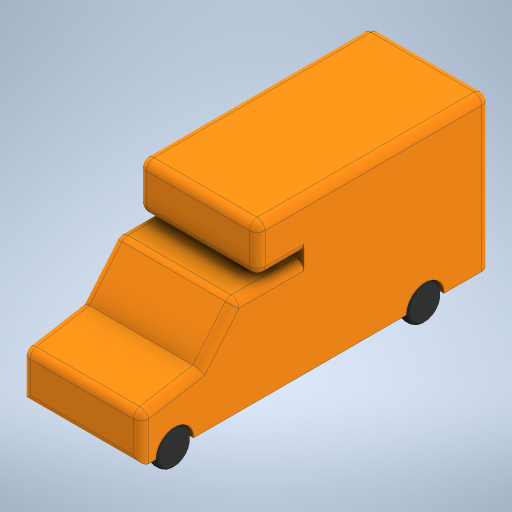
# Autodesk Inventor part: BungaCamp-Uhaul15ft
Saved by Autodesk Inventor 2023 (Build 270158000, 158)
## iProperties
Created: 2024-07-15
Part Number: BungaCamp-Uhaul15ft
Material: Generic
Document SubType Name: Modeling
Designer: incep
Density: 1 g/cm^3
Appearance: Default
Author: incep
Autodesk Inventor part; units mm, degrees
ref_plane "YZ Plane" through (0, 0, 0) normal (1, 0, 0) x (0, 1, 0)
ref_plane "XZ Plane" through (0, 0, 0) normal (0, 1, 0) x (-1, 0, 0)
ref_plane "XY Plane" through (0, 0, 0) normal (0, 0, 1) x (1, 0, 0)
sketch "Sketch4" plane through (0, 0, 0) normal (1, 0, 0) x (0, 1, 0)
  line L0 (2980.85, 1828.8) -> (0, 1828.8)
  line L1 (0, 1828.8) -> (0, -1828.8)
  line L2 (0, -1828.8) -> (2980.85, -1828.8)
  line L3 (2980.85, -1828.8) -> (2980.85, 1828.8)
  line L4 (2980.85, 2743.2) -> (2066.45, 2743.2)
  line L5 (2066.45, 2743.2) -> (2066.45, 1828.8)
  line L6 (2066.45, 1828.8) -> (2980.85, 1828.8)
  line L7 (2980.85, 1828.8) -> (2980.85, 2743.2)
  circle A0 centre (0, -558.8) radius 371.95
  line L8 (-371.95, 34.5004) -> (-371.95, -1152.1004) construction
  line L9 (0, 1828.8) -> (1914.05, 1828.8)
  line L10 (1914.05, 1828.8) -> (1914.05, 3174.9998)
  line L11 (1914.05, 3174.9998) -> (1096.7454, 3860.7998)
  line L12 (890.7249, 5029.1998) -> (1.7249, 5029.1998)
  line L13 (890.7249, 5029.1998) -> (1096.7454, 3860.7998)
  circle A1 centre (1.369, 4368.7999) radius 371.95
  line L14 (0, 1828.8) -> (1.7249, 5029.1998)
  point P0 (0, 0)
  point P1 (0, 0)
  point P2 (-371.95, -558.8)
  point P3 (1.5695, 4740.7498)
  point P4 (1.1685, 3996.8499)
  point P5 (0, -186.85)
  point P6 (0, -930.75)
  dimension "d2" = 4572
  dimension "d3" = 914.4
  dimension "d4" = 743.9
  dimension "d5" = 3352.8
  dimension "d6" = 914.4
  dimension "d7" = 6858
  dimension "d8" = 660.4
  dimension "d9" = 1270
  dimension "d10" = 152.4
  dimension "d11" = 130
  dimension "d12" = 100
  dimension "d13" = 889
  dimension "d14" = 685.8
  dimension "d15" = 1168.4
  constraints: 30 end point, 4 parallel, 3 horizontal, 2 centre point, 2 collinear, 2 midpoint, 2 perpendicular, 2 point on line, 1 coincident, 1 equal radius, 1 horizontal alignment, 1 tangent, 1 vertical
  measures "d2" distance between parallel lines of L2 L4
  measures "d3" distance of L4.start L4.end
  measures "d4" diameter of A0
  measures "d5" distance between parallel lines of L3 L8
  measures "d6" distance of L4.end L5.end
  measures "d7" distance of L1.end L12.end
  measures "d8" distance of A1.centre L12.end
  measures "d9" distance of L1.end A0.centre
  measures "d10" distance between parallel lines of L5 L10
  measures "d11" angle of L10 L11
  measures "d12" angle of L12 L13
  measures "d13" distance of L12.start L12.end
  measures "d14" vertical distance of L10.end L11.end
  measures "d15" vertical distance of L11.end L12.start
extrude "Extrusion1" add sketch "Sketch4" along normal mid plane 2336.8 contours L3 L2 L1 A0 L0 | L0 L5 L4 L7 | L0 L14 A1 L12 L13 L11 L10
sketch "Sketch5" plane through (1168.4, 0, 0) normal (1, 0, 0) x (0, 0, -1)
  circle A0 centre (-4368.7999, 1.369) radius 371.95 projected
  circle A1 centre (558.8, 0) radius 371.95 projected
  circle A2 centre (-4368.7999, 1.369) radius 346.55
  circle A3 centre (558.8, 0) radius 346.55
  point P0 (0, 0)
  dimension "d18" = 25.4
  dimension "d19" = 25.4
  constraints: 2 centre point
  measures "d18" radial gap between concentric circles of A0 A2
  measures "d19" radial gap between concentric circles of A1 A3
extrude "Extrusion2" add sketch "Sketch5" against normal blind 225 contours A2 | A3
sketch "Sketch6" plane through (-1168.4, 0, 0) normal (-1, 0, 0) x (0, 0, 1)
  circle A0 centre (-558.8, 0) radius 371.95 projected
  circle A1 centre (4368.7999, 1.369) radius 371.95 projected
  circle A2 centre (-558.8, 0) radius 346.55
  circle A3 centre (4368.7999, 1.369) radius 346.55
  point P0 (0, 0)
  dimension "d22" = 25.4
  dimension "d23" = 25.4
  constraints: 2 centre point
  measures "d22" radial gap between concentric circles of A0 A2
  measures "d23" radial gap between concentric circles of A1 A3
extrude "Extrusion3" add sketch "Sketch6" against normal blind 225 contours A2 | A3
fillet "Fillet1" radius 152.4 22 edges at (1168.4, 446.2249, 5029.1998) (-1168.4, 446.2249, 5029.1998) (-1168.4, 993.7352, 4444.9998) (1168.4, 993.7352, 4444.9998) (1168.4, 1505.3977, 3517.8998) (-1168.4, 1505.3977, 3517.8998) (0, 1914.05, 3174.9998) (1168.4, 2523.65, 2743.2) (-1168.4, 2523.65, 2743.2) (0, 2980.85, 2743.2) (0, 2066.45, 2743.2) (1168.4, 1914.05, 2501.8999) (-1168.4, 1914.05, 2501.8999) (0, 890.7249, 5029.1998) (1168.4, 2980.85, 457.2) (0, 2980.85, -1828.8) (-1168.4, 2980.85, 457.2) (1168.4, 1490.425, -1828.8) (-1168.4, 1490.425, -1828.8) (-1168.4, 2066.45, 2286) (1168.4, 2066.45, 2286) (0, 1.7249, 5029.1998)
fillet "Fillet2" radius 76.2 8 edges at (-1168.4, 0, -905.35) (-943.4, 0, -905.35) (943.4, 0, -212.25) (1168.4, 0, -212.25) (-1168.4, 1.369, 4022.2499) (-943.4, 1.369, 4022.2499) (943.4, 1.369, 4715.3499) (1168.4, 1.369, 4715.3499)
body "Solid1"
